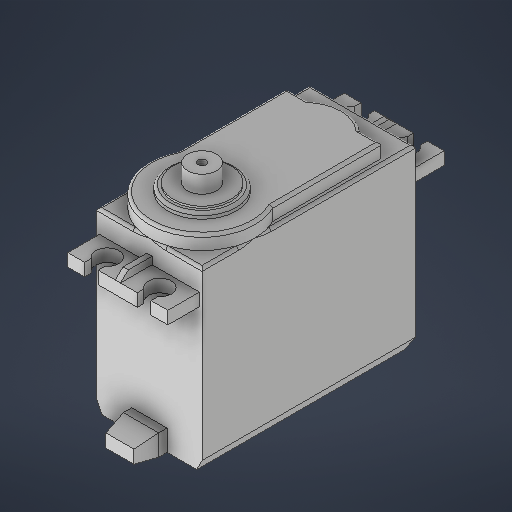
# Autodesk Inventor part: MMAE 232 CAD Assignment 2 Servo-Nicholas Skiba
Saved by Autodesk Inventor 2026.1 (Build 301233000, 233)
## iProperties
Created: 2025-08-28
Part Number: MMAE 232 CAD Assignment 2 Servo-Nicholas Skiba
Material: Generic
Document SubType Name: Modeling
Designer: Nick
Density: 1 g/cm^3
Appearance: Default
Author: Nick
Autodesk Inventor part; units mm, degrees
ref_plane "YZ Plane" through (0, 0, 0) normal (1, 0, 0) x (0, 1, 0)
ref_plane "XZ Plane" through (0, 0, 0) normal (0, 1, 0) x (-1, 0, 0)
sketch "Sketch1" plane through (0, 0, 0) normal (0, 1, 0) x (-1, 0, 0)
  line L0 (0, 0) -> (20, 0)
  line L1 (20, 0) -> (20, -40.5)
  line L2 (20, -40.5) -> (0, -40.5)
  line L3 (0, -40.5) -> (0, 0)
  dimension "d0" = 20
  dimension "d1" = 40.5
  constraints: 8 end point, 2 parallel, 1 horizontal, 1 perpendicular
  measures "d0" distance of L1.end L2.end
  measures "d1" distance of L0.end L1.end
extrude "Extrusion1" add sketch "Sketch1" along normal blind 33.6
sketch "Sketch2" plane through (-20, 0, 0) normal (0, 0, 1) x (1, 0, 0)
  line L0 (20, 0) -> (0, 0) projected
  line L1 (0, 0) -> (6.65, 0)
  line L2 (6.65, 0) -> (13.35, 0)
  line L3 (13.35, 0) -> (13.35, 4)
  line L4 (13.35, 4) -> (6.65, 4)
  line L5 (6.65, 4) -> (6.65, 0)
  dimension "d4" = 6.65
  dimension "d5" = 6.7
  dimension "d6" = 4
  constraints: 10 end point, 2 parallel, 1 horizontal, 1 perpendicular, 1 point on line
  measures "d4" distance of L0.end L1.end
  measures "d5" distance of L4.end L3.end
  measures "d6" distance of L3.end L2.end
extrude "Extrusion2" add sketch "Sketch2" along normal blind 1.6
sketch "Sketch3" plane through (-20, 0, 1.6) normal (0, 0, 1) x (1, 0, 0)
  line L0 (6.65, 0) -> (13.35, 0) projected
  line L1 (6.65, 0) -> (6.65, 0.5)
  line L2 (6.65, 4) -> (6.65, 0) projected
  line L3 (6.65, 0) -> (7.35, 0)
  line L4 (7.35, 0) -> (7.35, 0.5)
  line L5 (7.35, 0.5) -> (6.65, 0.5)
  line L6 (6.65, 0.5) -> (6.65, 0)
  line L7 (7.35, 0.5) -> (12.65, 0.5)
  line L8 (12.65, 0.5) -> (12.65, 3)
  line L9 (12.65, 3) -> (7.35, 3)
  line L10 (7.35, 3) -> (7.35, 0.5)
  point P0 (20, 0)
  dimension "d9" = 0.5
  dimension "d10" = 0.7
  dimension "d11" = 0.5
  dimension "d12" = 5.3
  dimension "d13" = 2.5
  constraints: 18 end point, 4 parallel, 2 horizontal, 2 perpendicular, 1 point on line
  measures "d9" distance of L0.start L1.end
  measures "d10" distance of L5.end L4.end
  measures "d11" distance of L4.end L3.end
  measures "d12" distance of L9.end L8.end
  measures "d13" distance of L8.end L7.end
extrude "Extrusion3" add sketch "Sketch3" along normal blind 4 contours L10 L9 L8 L7
loft "Loft1" add section 1 edges at (-13.35, 2, 1.6) (-10, 0, 1.6) (-6.65, 2, 1.6) (-10, 4, 1.6) section 2 edges at (-7.35, 1.75, 5.6) (-10, 3, 5.6) (-12.65, 1.75, 5.6) (-10, 0.5, 5.6)
chamfer "Chamfer1" distance 1 angle 63.4 3 edges at (0, 0, -20.25) (-10, 0, -40.5) (-20, 0, -20.25) measured on face at (-0.5, 0, -20.25) measured on face at (-19.5, 0, -20.25) measured on face at (-10, 0, -40)
sketch "Sketch4" plane through (-20, 33.6, 0) normal (0, 0, 1) x (1, 0, 0)
  line L0 (0, -31.603046) -> (0, 0)
  line L1 (0, 0) -> (0.5, 0)
  line L2 (0.5, 0) -> (0.5, -4.15)
  line L3 (0.5, -4.15) -> (0, -4.15)
  line L4 (0, -4.15) -> (0, 0)
  line L5 (0.5, -4.15) -> (19.5, -4.15)
  line L6 (19.5, -4.15) -> (19.5, -6.55)
  line L7 (19.5, -6.55) -> (0.5, -6.55)
  line L8 (0.5, -6.55) -> (0.5, -4.15)
  point P0 (20, -33.6)
  dimension "d23" = 0.5
  dimension "d24" = 4.15
  dimension "d25" = 19
  dimension "d26" = 2.4
  constraints: 16 end point, 4 parallel, 2 horizontal, 2 perpendicular
  measures "d23" distance of L2.end L3.end
  measures "d24" distance of L1.end L2.end
  measures "d25" distance of L6.end L7.end
  measures "d26" distance of L5.end L6.end
extrude "Extrusion4" add sketch "Sketch4" along normal blind 6 contours L5 L6 L7 L8
sketch "Sketch5" plane through (-19.5, 29.45, 0) normal (0, 1, 0) x (1, 0, 0)
  line L0 (-0.5, 0) -> (19.5, 0)
  line L1 (9.5, 0) -> (9.5, -6)
  line L2 (0, -6) -> (19, -6)
  line L3 (9.5, -6) -> (9, -6)
  line L4 (9, -6) -> (10, -6)
  line L5 (10, -6) -> (10, 0)
  line L6 (10, 0) -> (9, 0)
  line L7 (9, 0) -> (9, -6)
  line L8 (19, -6) -> (15.8, -6)
  line L9 (15.8, -6) -> (15.8, -4.5)
  line L10 (15.8, -4.5) -> (15.8, -3) construction
  line L11 (15.8, -3) -> (14.5, -3) construction
  arc A0 (15.8, -4.749971) -> (13.2, -4.749971) centre (14.5, -3) ccw
  line L12 (15.8, -4.749971) -> (13.2, -4.749971) construction
  line L13 (13.2, -4.749971) -> (13.2, -6)
  line L14 (13.2, -6) -> (15.8, -6)
  line L15 (19, -6) -> (0, -6)
  line L16 (3.2, -6) -> (3.2, -4.5)
  arc A1 (5.8, -4.749971) -> (3.2, -4.749971) centre (4.5, -3) ccw
  line L17 (5.8, -4.749971) -> (5.8, -6)
  line L18 (5.8, -6) -> (3.2, -6)
  point P0 (9, 0)
  dimension "d29" = 0.5
  dimension "d30" = 1
  dimension "d31" = 6
  dimension "d32" = 3.2
  dimension "d33" = 1.5
  dimension "d34" = 1.5
  dimension "d35" = 1.3
  dimension "d36" = 4.36
  constraints: 34 end point, 8 point on line, 8 symmetric about line, 5 perpendicular, 4 point on circle, 2 centre point, 2 midpoint, 2 parallel, 1 coincident, 1 collinear, 1 horizontal, 1 other
  measures "d29" distance of L1.end L3.end
  measures "d30" distance of L6.end L5.end
  measures "d31" distance of L5.end L4.end
  measures "d32" distance of L2.end L8.end
  measures "d33" distance of L8.end L9.end
  measures "d34" distance of L9.end L10.end
  measures "d35" distance of L10.end L11.end
  measures "d36" diameter of A0
extrude "Extrusion5" cut sketch "Sketch5" against normal blind 6 contours L16 A1 L17 L2 | L13 A0 L9 L2
extrude "Extrusion6" add sketch "Sketch5" along normal blind 1.4 contours L0 L1 L2 L7 | L0 L5 L2 L1
sketch "Sketch6" plane through (-9.5, 29.45, 6) normal (1, 0, 0) x (0, 0, -1)
  line L0 (0, 0) -> (0, 1.4) projected
  line L1 (0, 0) -> (0, 1.4)
  line L2 (0, 1.4) -> (1.5, 1.4)
  line L3 (0, 1.4) -> (6, 1.4) projected
  line L4 (1.5, 1.4) -> (0, 0)
  point P0 (6, -29.45)
  dimension "d41" = 1.5
  constraints: 6 end point, 1 point on line, 1 vertical
  measures "d41" distance of L0.end L2.end
extrude "Extrusion7" cut sketch "Sketch6" against normal blind 1.4
ref_plane "Work Plane1" through (-20, 33.6, -20.25) normal (0, 0, 1) x (1, 0, 0)
mirror "Mirror1" about plane through (-20, 33.6, -20.25) normal (0, 0, 1) of "Extrusion4", "Extrusion5", "Extrusion7", "Extrusion6"
sketch "Sketch7" plane through (0, 33.6, 0) normal (0, 1, 0) x (1, 0, 0)
  line L0 (-0.5, 0) -> (-19.5, 0)
  line L1 (-10, 0) -> (-10, 10)
  arc A0 (-18.93, 14.500567) -> (-0.535, 13.227038) centre (-10, 10) ccw
  line L2 (-20, 40.5) -> (-20, 0)
  line L3 (-20, 0) -> (-20, 35)
  line L4 (-20, 35) -> (-18.93, 35)
  line L5 (-18.93, 35) -> (-18.93, 14.500567)
  line L6 (-10, 0) -> (-10, 29.48)
  arc A1 (-5.071552, 35) -> (-14.928448, 35) centre (-10, 29.48) ccw
  line L7 (-18.93, 35) -> (-14.928448, 35)
  line L8 (-5.071552, 35) -> (-1.07, 35)
  line L9 (-1.07, 35) -> (-1, 14.358899)
  line L10 (-1, 0) -> (-1, 39.5)
  arc A2 (-18.93, 14.500567) -> (-1, 14.358899) centre (-10, 10) ccw
  line L11 (0, 40.5) -> (-20, 40.5)
  point P0 (0, 0)
  point P1 (-20, 10)
  dimension "d45" = 10
  dimension "d46" = 35
  dimension "d47" = 1.07
  dimension "d48" = 17.86
  dimension "d49" = 29.48
  dimension "d50" = 14.8
  dimension "d73" = 0
  dimension "d74" = 0
  constraints: 16 end point, 7 point on circle, 3 centre point, 3 coincident, 3 point on line, 2 vertical, 1 midpoint, 1 perpendicular
  measures "d45" distance of L1.start L1.end
  measures "d46" distance of L2.end L3.end
  measures "d47" distance of L3.end L4.end
  measures "d48" distance of L4.end L8.end
  measures "d49" distance of L1.start L6.end
  measures "d50" diameter of A1
  measures "d73" angle of L11 L7
  measures "d74" angle of L11 L8
extrude "Extrusion8" add sketch "Sketch7" along normal blind 2.68 contours A0 L5 L7 A1 L8 L9 L10 | L10 A2 A0
sketch "Sketch8" plane through (0, 36.28, 0) normal (0, 1, 0) x (1, 0, 0)
  line L0 (-10.5, 0) -> (-9.5, 0) projected
  line L1 (-10, 0) -> (-10, 10)
  circle A0 centre (-10, 10) radius 6.5
  circle A1 centre (-10, 10) radius 5.5
  circle A2 centre (-10, 10) radius 2.75
  point P0 (0, 0)
  dimension "d53" = 10
  dimension "d54" = 13
  dimension "d55" = 11
  dimension "d56" = 5.5
  constraints: 3 centre point, 3 coincident, 2 end point, 1 midpoint, 1 vertical
  measures "d53" distance of L1.start L1.end
  measures "d54" diameter of A0
  measures "d55" diameter of A1
  measures "d56" diameter of A2
extrude "Extrusion9" add sketch "Sketch8" along normal blind 1.1 contours A0
extrude "Extrusion10" add sketch "Sketch8" along normal blind 1.45 contours A1
extrude "Extrusion11" add sketch "Sketch8" along normal blind 4.75 contours A2
sketch "Sketch9" plane through (-10, 41.03, -10) normal (0, 1, 0) x (1, 0, 0)
  line L0 (10, 0) -> (10, 30.5) projected
  line L1 (-10, -10) -> (0, -10) projected
  point P0 (10, -10)
  point P1 (0, 0)
  dimension "d63" = 10
  dimension "d64" = 10
  measures "d63" distance from line of L0 point (0, 0)
  measures "d64" distance from line of L1 point (0, 0)
hole "Hole1" at (-10, 41.03, -10) direction (0, -1, 0) diameter 1.567 depth 8 tip angle 118 thread size "M2x0.4" class "6H" standard "ANSI Metric M Profile"
fillet "Fillet1" radius 0.5 8 edges at (-16.5, 37.38, -10) (0, 33.6, -5) (0, 33.6, -25.25) (-5, 33.6, 0) (-15, 33.6, 0) (-20, 33.6, -5) (-20, 33.6, -25.25) (-10, 33.6, -40.5)
fillet "Fillet2" radius 0.5 3 edges at (-10, 36.28, -36.88) (-3.0708, 36.28, -35) (-1.035, 36.28, -24.6794)
fillet "Fillet3" radius 0.5 5 edges at (-14.5342, 36.28, -35) (-16.9292, 36.28, -35) (-18.93, 36.28, -24.7503) (-10.079, 36.28, -0.0003) (-1.2396, 36.28, -14.8224)
body "Solid1"
